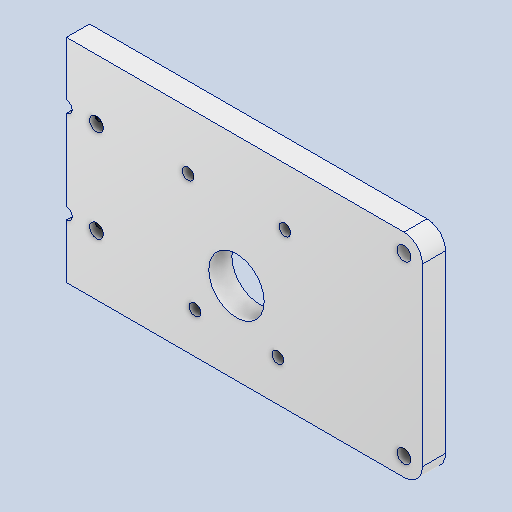
# Autodesk Inventor part: odom_v1_Plate_3
Saved by Autodesk Inventor 2025.2 (Build 292293000, 293)
## iProperties
Created: 2025-03-30
Part Number: odom_v1_Plate_3
Material: アルミニウム 6061
Document SubType Name: Modeling
Designer: haruy
Density: 2.7 g/cm^3
Appearance: アルミニウム - フラット
Author: haruy
Autodesk Inventor part; units mm, degrees
ref_plane "YZ Plane" through (0, 0, 0) normal (1, 0, 0) x (0, 1, 0)
ref_plane "XZ Plane" through (0, 0, 0) normal (0, 1, 0) x (-1, 0, 0)
ref_plane "XY Plane" through (0, 0, 0) normal (0, 0, 1) x (1, 0, 0)
derived "odom_v1_Sketch_Base.ipt"
sketch "スケッチ2" plane through (0, 0, -300) normal (0, 0, 1) x (1, 0, 0)
  line L0 (0, 0) -> (-20, 0) projected
  line L1 (-20, 0) -> (-20, 20) projected
  line L2 (-20, 20) -> (0, 20) projected
  line L3 (0, 20) -> (0, 0) projected
  line L4 (223.462, -77) -> (-136.7068, -77) projected
  line L5 (5, -2) -> (10.5, -2) projected
  line L6 (10.5, -2) -> (10.5, -57) projected
  line L7 (10.5, -57) -> (5, -57) projected
  line L8 (5, -57) -> (5, -2) projected
  line L9 (10.5, -52) -> (15, -52) projected
  line L10 (15, -52) -> (15, -22) projected
  line L11 (15, -22) -> (10.5, -22) projected
  line L12 (10.5, -22) -> (10.5, -52) projected
  line L13 (15, -66) -> (20, -66) projected
  line L14 (20, -66) -> (20, -20) projected
  line L15 (20, -20) -> (15, -20) projected
  line L16 (15, -20) -> (15, -66) projected
  circle A0 centre (56.8145, -48.1855) radius 28.8145 projected
  circle A1 centre (22, 48) radius 1.65 projected
  circle A2 centre (22, -17) radius 1.65 projected
  line L17 (22, 48) -> (22, -17) projected
  line L18 (71.2015, -63.5145) -> (42.4265, -63.5145) projected
  line L19 (42.4265, -63.5145) -> (42.4265, -20.1385) projected
  line L20 (42.4265, -20.1385) -> (71.2015, -20.1385) projected
  line L21 (71.2015, -20.1385) -> (71.2015, -63.5145) projected
  line L22 (30.5, -12) -> (13.5, -12) projected
  line L23 (13.5, -12) -> (13.5, 33.5) projected
  line L24 (13.5, 33.5) -> (30.5, 33.5) projected
  line L25 (30.5, 33.5) -> (30.5, -12) projected
  circle A3 centre (93.0874, -24) radius 4 projected
  circle A4 centre (93.0874, -62) radius 4 projected
  line L26 (93.0874, -24) -> (93.0874, -62) projected
  line L27 (93.0874, -66) -> (20, -66) projected
  line L28 (97.0874, -24) -> (97.0874, -62) projected
  line L29 (93.0874, -20) -> (20, -20) projected
  circle A5 centre (93.0874, -24) radius 1.5
  circle A6 centre (93.0874, -62) radius 1.5
  circle A7 centre (56.8145, -48.1855) radius 6
  circle A8 centre (65.7935, -57.1655) radius 1.25
  line L30 (56.814, -63.5145) -> (56.814, -20.1385)
  circle A9 centre (67.2915, -32.4375) radius 1.25
  circle A10 centre (47.8345, -57.1655) radius 1.25
  circle A11 centre (46.3365, -32.4375) radius 1.25
  line L31 (24, -12) -> (20, -12) projected
  line L32 (20, -12) -> (20, -20) projected
  line L33 (20, -20) -> (24, -20) projected
  line L34 (24, -20) -> (24, -12) projected
  circle A12 centre (26.5, -53) radius 1.5
  circle A13 centre (26.5, -33) radius 1.5
  circle A14 centre (20, -33) radius 1.25
  circle A15 centre (20, -53) radius 1.25
  point P0 (25, -55.4336)
  point P1 (30.1534, -56)
  point P2 (22, -12)
  point P3 (22, 33.5)
  point P4 (33.5, -32.8395)
  point P5 (33.5, -20)
  point P6 (20, -56)
  point P7 (34.1668, -66)
  point P8 (79.4622, -66)
  point P9 (62.8022, -20)
  point P10 (50.8268, -20)
  point P11 (20, -31.75)
  point P12 (20, -34.25)
  point P13 (20, -51.75)
  point P14 (20, -54.25)
  dimension "d1" = 3
  dimension "d2" = 3
  dimension "d3" = 12
  dimension "d4" = 2.5
  dimension "d5" = 6.349
  dimension "d6" = 5.408
  dimension "d7" = 2.5
  dimension "d8" = 12.299
  dimension "d9" = 3.91
  dimension "d23" = 3
  dimension "d24" = 3
  dimension "d25" = 13
  dimension "d26" = 20
  dimension "d27" = 6.5
  dimension "d28" = 6.5
  dimension "d29" = 2.5
  dimension "d30" = 2.5
  dimension "d31" = 13
  dimension "d32" = 20
  constraints: 11 centre point, 3 coincident, 2 end point, 2 midpoint, 2 point on line, 2 symmetric about line, 2 other
  measures "d1" diameter of A5
  measures "d2" diameter of A6
  measures "d3" diameter of A7
  measures "d4" diameter of A8
  measures "d5" distance from line of A8.centre L18
  measures "d6" distance from line of A8.centre L21
  measures "d7" diameter of A9
  measures "d8" distance from line of L20 A9.centre
  measures "d9" distance from line of A9.centre L21
  measures "d23" diameter of A12
  measures "d24" diameter of A13
  measures "d25" distance from line of A12.centre L27
  measures "d26" distance of A13.centre A12.centre
  measures "d27" distance from line of A12.centre L14
  measures "d28" distance from line of A13.centre L14
  measures "d29" diameter of A14
  measures "d30" diameter of A15
  measures "d31" distance from line of A15.centre L27
  measures "d32" distance of A14.centre A15.centre
extrude "押し出し1" add sketch "スケッチ2" along normal blind 5 contours L29 A0 L20 L19 L27 L14 A15 A14 | A0 L19 L18 L21 L27 | L29 A0 L20 | L19 L20 A0 | A0 L20 L30 A7 L18 L19 | A0 L21 L20 L29 A3 L26 A4 L27 | A4 | L20 L21 A0 | A0 L21 L18 L30 A7 L20 | A3 | A4 L26 A3 L28
sketch "スケッチ3" plane through (20, -66, -300) normal (-1, 0, 0) x (0, 0, 1)
  line L0 (0, 46) -> (0, 0) projected
  line L1 (0, 0) -> (5, 0) projected
  point P0 (300, 66)
  point P1 (2.5, 33)
  point P2 (2.5, 13)
  point P3 (0, 10)
  dimension "d12" = 2.5
  dimension "d13" = 2.5
  dimension "d14" = 13
  dimension "d15" = 20
  measures "d12" distance from line of point (2.5, 13) L0
  measures "d13" distance from line of point (2.5, 33) L0
  measures "d14" distance from line of point (2.5, 13) L1
  measures "d15" distance of point (2.5, 33) point (2.5, 13)
hole "穴1" at (20, -33, -297.5) at (20, -53, -297.5) direction (1, 0, 0) diameter 2.5 depth 10 tip angle 118
equation "\"d2\" = d1"
equation "\"d28\" = d27"
equation "\"d30\" = d29"
equation "\"d31\" = d25"
equation "\"d32\" = d26"
equation "\"d13\" = d12"
